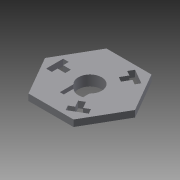
# Autodesk Inventor part: Base
Saved by Autodesk Inventor 2014 SP1 (Build 180222100, 222)
## iProperties
Created: 2013-10-27
Part Number: Base
Material: Genérico
Document SubType Name: Modeling
Designer: Gregorio
Density: 1 g/cm^3
Appearance: Valor por defecto
Author: Gregorio
Autodesk Inventor part; units mm, degrees
ref_plane "YZ Plane" through (0, 0, 0) normal (1, 0, 0) x (0, 1, 0)
ref_plane "XZ Plane" through (0, 0, 0) normal (0, 1, 0) x (-1, 0, 0)
ref_plane "XY Plane" through (0, 0, 0) normal (0, 0, 1) x (1, 0, 0)
sketch "Boceto1" plane through (0, 0, 0) normal (0, 0, 1) x (1, 0, 0)
  line L0 (17.3205, 30) -> (34.641, 0)
  line L1 (34.641, 0) -> (17.3205, -30)
  line L2 (17.3205, -30) -> (-17.3205, -30)
  line L3 (-17.3205, -30) -> (-34.641, 0)
  line L4 (-34.641, 0) -> (-17.3205, 30)
  line L5 (-17.3205, 30) -> (17.3205, 30)
  point P0 (0, 0)
  point P1 (0, 0)
  dimension "d0" = 30
  constraints: 12 end point, 1 coincident, 13 other
  measures "d0" distance from line of L5 point (0, 0)
extrude "Extrusión1" add sketch "Boceto1" along normal blind 5
sketch "Boceto3" plane through (0, 0, 5) normal (0, 0, 1) x (1, 0, 0)
  circle A0 centre (0, 0) radius 9
  dimension "d5" = 18
  constraints: 1 centre point, 1 coincident
  measures "d5" diameter of A0
extrude "Extrusión3" cut sketch "Boceto3" against normal blind 10
sketch "Boceto4" plane through (0, 0, 5) normal (0, 0, 1) x (1, 0, 0)
  circle A0 centre (0, 0) radius 9 projected
  line L0 (-6.15, 6.571) -> (6.15, 6.571)
  line L1 (6.15, 6.571) -> (6.15, -17.029)
  line L2 (6.15, -17.029) -> (-6.15, -17.029)
  line L3 (-6.15, -17.029) -> (-6.15, 6.571)
  point P0 (0, 6.571)
  dimension "d10" = 12.3
  dimension "d11" = 23.6
  constraints: 8 end point, 2 parallel, 1 horizontal, 1 midpoint, 1 perpendicular, 1 vertical alignment, 2 other
  measures "d10" distance of L1.end L2.end
  measures "d11" distance of L0.end L1.end
extrude "Extrusión4" cut sketch "Boceto4" against normal blind 3 contours L1 A0 L3 L0 | L1 L2 L3 A0
sketch "Boceto5" plane through (0, 0, 5) normal (0, 0, 1) x (1, 0, 0)
  line L0 (6.15, -17.029) -> (-6.15, -17.029) projected
  line L1 (34.641, 0) -> (17.3205, 30) projected
  line L2 (-34.641, 0) -> (-17.3205, -30) projected
  line L3 (-17.3205, -30) -> (17.3205, -30) projected
  line L4 (17.3205, -30) -> (34.641, 0) projected
  line L5 (6.5197, 15.6925) -> (11.6697, 24.6126)
  line L6 (11.6697, 24.6126) -> (15.4803, 22.4126)
  line L7 (15.4803, 22.4126) -> (10.3303, 13.4925)
  line L8 (10.3303, 13.4925) -> (6.5197, 15.6925)
  line L9 (6.5197, 15.6925) -> (15.4803, 22.4126) construction
  line L10 (11.6697, 24.6126) -> (10.3303, 13.4925) construction
  line L11 (-16.85, -2.2) -> (-27.15, -2.2)
  line L12 (-27.15, -2.2) -> (-27.15, 2.2)
  line L13 (-27.15, 2.2) -> (-16.85, 2.2)
  line L14 (-16.85, 2.2) -> (-16.85, -2.2)
  line L15 (-16.85, -2.2) -> (-27.15, 2.2) construction
  line L16 (-27.15, -2.2) -> (-16.85, 2.2) construction
  line L17 (6.5197, -15.6925) -> (11.6697, -24.6126)
  line L18 (11.6697, -24.6126) -> (15.4803, -22.4126)
  line L19 (15.4803, -22.4126) -> (10.3303, -13.4925)
  line L20 (10.3303, -13.4925) -> (6.5197, -15.6925)
  line L21 (6.5197, -15.6925) -> (15.4803, -22.4126) construction
  line L22 (11.6697, -24.6126) -> (10.3303, -13.4925) construction
  arc A0 (6.15, -6.571) -> (-6.15, -6.571) centre (0, 0) ccw projected
  line L23 (-17.3205, 30) -> (-34.641, 0) projected
  line L24 (0, 0) -> (17.3205, 30)
  line L25 (0, 0) -> (17.3205, -30)
  line L26 (-27.15, -2.2) -> (-22.85, -2.2)
  line L27 (-27.15, -2.2) -> (-22.75, -2.2)
  line L28 (-22.75, -2.2) -> (-22.75, -6.6)
  line L29 (-22.75, -6.6) -> (-27.15, -6.6)
  line L30 (-27.15, -6.6) -> (-27.15, -2.2)
  line L31 (15.4803, -22.4126) -> (13.2803, -18.6021)
  line L32 (13.2803, -18.6021) -> (17.0908, -16.4021)
  line L33 (17.0908, -16.4021) -> (19.2908, -20.2126)
  line L34 (19.2908, -20.2126) -> (15.4803, -22.4126)
  line L35 (11.6697, 24.6126) -> (9.4697, 20.8021)
  line L36 (9.4697, 20.8021) -> (5.6592, 23.0021)
  line L37 (5.6592, 23.0021) -> (7.8592, 26.8126)
  line L38 (7.8592, 26.8126) -> (11.6697, 24.6126)
  line L39 (15.4803, 22.4126) -> (19.2908, 20.2126)
  line L40 (19.2908, 20.2126) -> (17.4071, 16.95)
  line L41 (17.4071, 16.95) -> (13.5966, 19.15)
  line L42 (13.5966, 19.15) -> (15.4803, 22.4126)
  line L43 (11.6697, -24.6126) -> (8.0324, -26.7126)
  line L44 (8.0324, -26.7126) -> (5.8324, -22.9021)
  line L45 (5.8324, -22.9021) -> (9.4697, -20.8021)
  line L46 (9.4697, -20.8021) -> (11.6697, -24.6126)
  line L47 (-27.15, 2.2) -> (-27.15, 6.5)
  line L48 (-27.15, 6.5) -> (-22.85, 6.5)
  line L49 (-22.85, 6.5) -> (-22.85, 2.2)
  line L50 (-22.85, 2.2) -> (-27.15, 2.2)
  point P0 (11, 19.0526)
  point P1 (-22, 0)
  point P2 (11, -19.0526)
  point P3 (-22, 0)
  point P4 (-22, 0)
  point P5 (12.5, 21.6506)
  point P6 (13.575, 23.5126)
  point P7 (11, 19.0526)
  point P8 (11, -19.0526)
  point P9 (12.5, -21.6506)
  point P10 (-27.15, 0)
  point P11 (13.575, -23.5126)
  dimension "d16" = 4.4
  dimension "d17" = 10.3
  dimension "d18" = 4.4
  dimension "d20" = 4.4
  dimension "d21" = 10.3
  dimension "d47" = 22
  dimension "d48" = 22
  dimension "d49" = 22
  dimension "d60" = 4.4
  dimension "d61" = 4.4
  dimension "d62" = 4.4
  dimension "d63" = 4.4
  dimension "d64" = 4.4
  dimension "d65" = 4.4
  dimension "d68" = 4.4
  dimension "d69" = 4.4
  dimension "d70" = 4.3
  constraints: 90 end point, 24 parallel, 12 midpoint, 10 perpendicular, 6 point on line, 3 collinear, 2 horizontal, 1 horizontal alignment
  measures "d16" distance of L5.end L6.end
  measures "d17" distance of L6.end L7.end
  measures "d18" distance of L11.end L12.end
  measures "d20" distance of L18.end L17.end
  measures "d21" distance of L18.end L19.end
  measures "d47" distance of L24.start point (-22, 0)
  measures "d48" distance of point (11, 19.053) L24.start
  measures "d49" distance of L24.start point (11, -19.053)
  measures "d60" distance of L28.end L29.end
  measures "d61" distance of L27.end L28.end
  measures "d62" distance of L18.end L31.end
  measures "d63" distance of L31.end L32.end
  measures "d64" distance of L5.end L35.end
  measures "d65" distance of L35.end L36.end
  measures "d68" distance of L6.end L39.end
  measures "d69" distance of L43.end L44.end
  measures "d70" distance of L12.end L47.end
sketch "Boceto9" plane through (0, 0, 0) normal (0, 0, -1) x (-1, 0, 0)
  circle A0 centre (0, 0) radius 9 projected
  circle A1 centre (0, 0) radius 12
  circle A2 centre (0, 0) radius 9
  constraints: 2 centre point, 2 coincident, 1 concentric
extrude "Extrusión9" add sketch "Boceto9" along normal blind 3
extrude "Extrusión11" cut sketch "Boceto5" against normal blind 10 contours L24 L8 L5 L6 | L6 L7 L8 L24 | L25 L20 L19 L18 | L18 L17 L20 L25 | L5 L36 L37 L38 | L39 L40 L41 L7 | L43 L44 L45 L17 | L19 L32 L33 L34 | L11 L12 L13 L14 | L28 L29 L30 L11 | L13 L47 L48 L49
